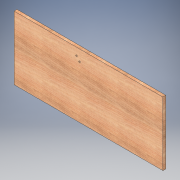
# Autodesk Inventor part: Grundplatte
Saved by Autodesk Inventor 2018 (Build 220112000, 112)
## iProperties
Created: 2018-03-14
Part Number: Grundplatte
Material: Holz (Birke)
Document SubType Name: Modeling
Designer: Julian
Density: 0.55 g/cm^3
Appearance: Birke - natur - poliert
Author: Julian
Autodesk Inventor part; units mm, degrees
ref_plane "YZ Plane" through (0, 0, 0) normal (1, 0, 0) x (0, 1, 0)
ref_plane "XZ Plane" through (0, 0, 0) normal (0, 1, 0) x (-1, 0, 0)
ref_plane "XY Plane" through (0, 0, 0) normal (0, 0, 1) x (1, 0, 0)
sketch "Skizze1" plane through (0, 0, 0) normal (0, 1, 0) x (-1, 0, 0)
  line L0 (0, 0) -> (-1000, 0)
  line L1 (-1000, 0) -> (-1000, 428)
  line L2 (-1000, 428) -> (0, 428)
  line L3 (0, 428) -> (0, 0)
  dimension "d0" = 1000
  dimension "d1" = 428
  constraints: 8 end point, 2 parallel, 1 horizontal, 1 perpendicular
  measures "d0" distance of L1.end L2.end
  measures "d1" distance of L0.end L1.end
extrude "Extrusion1" add sketch "Skizze1" along normal blind 20
sketch "Skizze2" plane through (0, 20, 0) normal (0, 1, 0) x (1, 0, 0)
  line L0 (0, 0) -> (0, -428) projected
  line L1 (0, -428) -> (220, -428)
  line L2 (220, -428) -> (220, -214)
  circle A0 centre (220, -214) radius 14
  dimension "d4" = 220
  dimension "d5" = 214
  dimension "d6" = 28
  constraints: 4 end point, 1 centre point, 1 coincident, 1 horizontal, 1 perpendicular
  measures "d4" distance of L0.end L1.end
  measures "d5" distance of L1.end L2.end
  measures "d6" diameter of A0
extrude "Extrusion2" cut sketch "Skizze2" against normal blind 11
sketch "Skizze3" plane through (0, 20, 0) normal (0, 1, 0) x (1, 0, 0)
  line L0 (0, -429.5296) -> (419.9972, -428)
  line L1 (0, -428) -> (1000, -428) projected
  line L2 (419.9972, -428) -> (419.8151, -378.0003)
  line L3 (419.8151, -378.0003) -> (439.815, -377.9275)
  line L4 (439.815, -377.9275) -> (439.7239, -352.9277)
  point P0 (0, 0)
  dimension "d9" = 420
  dimension "d10" = 50
  dimension "d11" = 20
  dimension "d12" = 25
  constraints: 8 end point, 3 perpendicular, 1 point on line
  measures "d9" distance of L0.start L0.end
  measures "d10" distance of L0.end L2.end
  measures "d11" distance of L2.end L3.end
  measures "d12" distance of L3.end L4.end
hole "Bohrung1" at (419.8151, 20, 378.0003) at (439.7239, 20, 352.9277) direction (0, -1, 0) diameter 10 depth 20 tip angle 118
